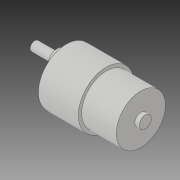
# Autodesk Inventor part: V-TEC 12V Mini 37D DC
Saved by Autodesk Inventor 2019.4 (Build 234330000, 330)
## iProperties
Part Number: V-TEC 12V Mini 37D DC
Material: Generisch
Document SubType Name: Modeling
Designer: rYan
Density: 1 g/cm^3
Appearance: Vorgabe
Author: rYan
Autodesk Inventor part; units mm, degrees
ref_plane "YZ Plane" through (0, 0, 0) normal (1, 0, 0) x (0, 1, 0)
ref_plane "XZ Plane" through (0, 0, 0) normal (0, 1, 0) x (-1, 0, 0)
ref_plane "XY Plane" through (0, 0, 0) normal (0, 0, 1) x (1, 0, 0)
sketch "Skizze1" plane through (0, 0, 0) normal (1, 0, 0) x (0, 1, 0)
  circle A0 centre (0, 0) radius 18.5
  dimension "d0" = 37
  constraints: 1 centre point, 1 coincident
  measures "d0" diameter of A0
extrude "Extrusion1" add sketch "Skizze1" along normal blind 26.5
sketch "Skizze2" plane through (26.5, 0, 0) normal (1, 0, 0) x (0, 0, -1)
  circle A0 centre (0, 0) radius 16.3
  dimension "d3" = 32.6
  constraints: 1 centre point, 1 coincident
  measures "d3" diameter of A0
extrude "Extrusion2" add sketch "Skizze2" along normal blind 23
sketch "Skizze3" plane through (49.5, 0, 0) normal (1, 0, 0) x (0, 0, -1)
  circle A0 centre (0, 0) radius 4
  dimension "d6" = 8
  constraints: 1 centre point, 1 coincident
  measures "d6" diameter of A0
extrude "Extrusion3" add sketch "Skizze3" along normal blind 3
sketch "Skizze4" plane through (0, 0, 0) normal (-1, 0, 0) x (0, 0, 1)
  line L0 (-25.9, 0) -> (25.9, 0) projected
  line L1 (0, 25.9) -> (0, -25.9) projected
  circle A0 centre (7, 0) radius 6
  point P0 (0, 0)
  dimension "d9" = 12
  dimension "d10" = 7
  constraints: 1 centre point, 1 point on line
  measures "d9" diameter of A0
  measures "d10" distance from line of L1 A0.centre
extrude "Extrusion4" add sketch "Skizze4" along normal blind 6
sketch "Skizze5" plane through (-6, 0, 7) normal (-1, 0, 0) x (0, 0, 1)
  circle A0 centre (0, 0) radius 6 projected
  circle A1 centre (0, 0) radius 3
  point P0 (-7, 0)
  dimension "d13" = 6
  constraints: 1 centre point, 1 coincident
  measures "d13" diameter of A1
extrude "Extrusion5" add sketch "Skizze5" along normal blind 15 contours A1
sketch "Skizze6" plane through (0, 0, 0) normal (-1, 0, 0) x (0, 0, 1)
  line L0 (-25.9, 0) -> (25.9, 0) projected
  line L1 (0, 25.9) -> (0, -25.9) projected
  circle A0 centre (0, 0) radius 15.4 construction
  point P0 (0, 15.4)
  point P1 (-13.3368, 7.7)
  point P2 (-13.3368, -7.7)
  point P3 (0, -15.4)
  point P4 (13.3368, -7.7)
  point P5 (13.3368, 7.7)
  dimension "d16" = 30.8
  dimension "d19" = 360
  constraints: 1 coincident, 1 point on line, 1 vertical alignment, 9 other
hole "Bohrung1" at (0, 15.4, 0) at (0, 7.7, -13.3368) at (0, -7.7, -13.3368) at (0, -15.4, 0) at (0, -7.7, 13.3368) at (0, 7.7, 13.3368) direction (1, 0, 0) diameter 2.459 depth 6 tip angle 118 thread size "M3x0.5" class "6H" standard "ISO Metric profile"
